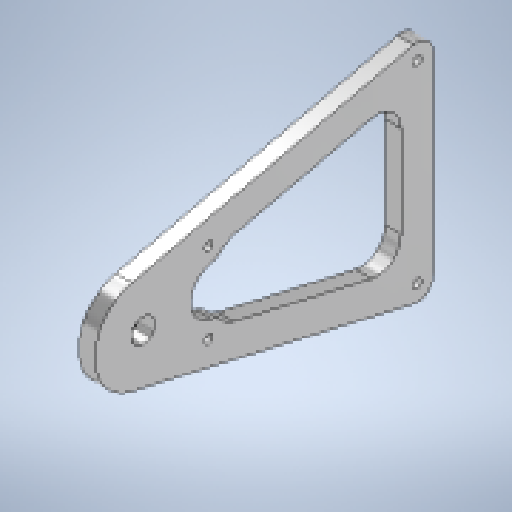
# Autodesk Inventor part: Frame (Motor Side)
Saved by Autodesk Inventor 2023.2 (Build 272271000, 271)
## iProperties
Created: 2022-05-22
Part Number: Frame (Motor Side)
Material: Aluminum 6061
Document SubType Name: Modeling
Designer: Nathan Cai
Density: 2.7 g/cm^3
Appearance: Aluminum - Flat
Mass: 78.0401 g
Surface Area: 132.733 cm^2
Volume: 28.9038 cm^3
Leg_Mounts: 0.625 in
Leg_Offset: 0.750 in
C2C: 4.263 in
Author: Nathan Cai
Autodesk Inventor part; units mm, degrees
ref_plane "YZ Plane" through (0, 0, 0) normal (1, 0, 0) x (0, 1, 0)
ref_plane "XZ Plane" through (0, 0, 0) normal (0, 1, 0) x (-1, 0, 0)
ref_plane "XY Plane" through (0, 0, 0) normal (0, 0, 1) x (1, 0, 0)
sketch "Sketch1" plane through (0, 0, 0) normal (1, 0, 0) x (0, 1, 0)
  circle A0 centre (0, 0) radius 4.7625 construction
  line L0 (0, 0) -> (0, 108.2802) construction
  circle A1 centre (0, 108.2802) radius 4.7625
  circle A2 centre (0, 108.2802) radius 76.2 construction
  circle A3 centre (0, 108.2802) radius 19.05
  line L1 (0, 0) -> (38.1, 0) construction
  circle A4 centre (38.1, 0) radius 1.7526
  circle A5 centre (38.1, 0) radius 6.35
  line L2 (18.5593, 112.5762) -> (44.2864, 1.432)
  line L3 (10.2367, 92.2144) -> (31.9136, -1.432)
  circle A6 centre (-38.1, 0) radius 1.7526
  circle A7 centre (-38.1, 0) radius 6.35
  line L4 (-18.5593, 112.5762) -> (-44.2864, 1.432)
  line L5 (-10.2367, 92.2144) -> (-31.9136, -1.432)
  line L6 (38.1, 6.35) -> (-38.1, 6.35)
  line L7 (-38.1, -6.35) -> (38.1, -6.35)
  line L8 (38.1, 0) -> (15.5749, 97.3109) construction
  circle A8 centre (19.05, 82.2982) radius 1.7526
  circle A9 centre (-19.05, 82.2982) radius 1.7526
  line L9 (19.05, 82.2982) -> (-19.05, 82.2982) construction
  circle A10 centre (15.875, 82.2982) radius 6.35
  circle A11 centre (15.875, 82.2982) radius 1.7526
  circle A12 centre (-15.875, 82.2982) radius 6.35
  circle A13 centre (-15.875, 82.2982) radius 1.7526
  arc A14 (31.7424, -0.6927) -> (-31.1085, -6.35) centre (0, 0) ccw construction
  arc A15 (44.45, 0) -> (-44.45, 0) centre (0, 0) ccw construction
  point P0 (44.2067, -1.741)
  point P1 (-22.5503, 39.0184)
  point P2 (-10.2367, 92.2144)
  point P3 (30.1122, 6.35)
  point P4 (-30.1122, 6.35)
  point P5 (-13.9314, 76.2529)
  point P6 (-11.4728, 86.8745)
  point P7 (11.4728, 86.8745)
  point P8 (13.9314, 76.2529)
  point P9 (22.7416, 38.1919)
  point P10 (-22.7416, 38.1919)
  point P11 (-40.254, 18.8525)
  point P12 (-44.3636, 7.3939)
  point P13 (-31.75, 0)
  point P14 (31.75, 0)
  point P15 (44.3636, 7.3939)
  point P16 (40.254, 18.8525)
  point P17 (-28.2095, 14.5701)
  point P18 (31.8736, 5.0775)
  point P19 (-31.7424, -0.6927)
  point P20 (28.2095, 14.5701)
  dimension "d0" = 9.525
  dimension "C2C" = 108.2802
  dimension "d3" = 9.525
  dimension "d4" = 152.4
  dimension "d5" = 38.1
  dimension "d6" = 38.1
  dimension "d7" = 3.5052
  dimension "d8" = 12.7
  dimension "d9" = 0
  dimension "d10" = 12.7
  dimension "d37" = 3.5052
  dimension "Leg_Offset" = 19.05
  dimension "d39" = 12.7
  dimension "d40" = 3.5052
  dimension "Leg_Mounts" = 15.875
  dimension "d42" = 12.7
  constraints: 20 end point, 18 point on circle, 16 centre point, 11 coincident, 10 symmetric about line, 7 tangent, 6 point on line, 2 horizontal, 2 parallel, 1 vertical, 5 other
  measures "d0" diameter of A0
  measures "C2C" distance of L0.start L0.end
  measures "d3" diameter of A1
  measures "d4" diameter of A2
  measures "d5" diameter of A3
  measures "d6" distance of L1.start L1.end
  measures "d7" diameter of A4
  measures "d8" diameter of A5
  measures "d9" distance from line of A0.centre L1
  measures "d10" distance between parallel lines of L2 L3
  measures "d37" diameter of A8
  measures "Leg_Offset" distance from line of L0 L9.start
  measures "d39" diameter of A10
  measures "d40" diameter of A11
  measures "Leg_Mounts" distance from line of L0 A11.centre
  measures "d42" radial gap between concentric circles of A14 A15
extrude "Extrusion1" add sketch "Sketch1" along normal blind 6.35 contours A3 | A3 L2 A5 L6 L3 A10 | A3 L5 A12 L6 A7 L4 | A5 | A10 L3 | L3 A10 | A7 | A5 L3 L6 | A12 L5 | L5 A12 | L6 L5 A7 | A7 L5 L6 L3 A5 L7 | A8 A11 | A13 A9 picked at (19.7267, 82.156) picked at (-19.7267, 82.4404)
fillet "Fillet1" radius 9.525 8 edges at (3.175, 10.2367, 92.2144) (3.175, -10.2367, 92.2144) (3.175, 13.9314, 76.2529) (3.175, -13.9314, 76.2529) (3.175, 11.4728, 86.8745) (3.175, -11.4728, 86.8745) (3.175, 30.1122, 6.35) (3.175, -30.1122, 6.35)
fillet "Fillet2" [suppressed]
equation "\"d10\" = d8"
body "Solid1"
